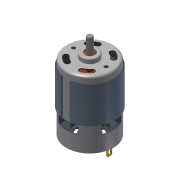
# Autodesk Inventor part: E Motor
Saved by Autodesk Inventor 2015 SP2 (Build 190223200, 223)
## iProperties
Created: 2015-09-01
Part Number: E Motor
Material: Iron, Cast
Document SubType Name: Modeling
Designer: Hassan
Density: 7.15 g/cm^3
Appearance: Iron Gray
Mass: 292.423 g
Surface Area: 270.91 cm^2
Volume: 40.8983 cm^3
Author: Hassan
Autodesk Inventor part; units mm, degrees
sketch "Sketch1" plane through (0, 0, 0) normal (0, 0, 1) x (1, 0, 0)
  circle A0 centre (0, 0) radius 21
  dimension "d3" = 42
  constraints: 1 centre point
  measures "d3" diameter of A0
extrude "Extrusion1" add sketch "Sketch1" along normal mid plane 59.5
sketch "Sketch2" plane through (0, 0, 29.75) normal (0, 0, 1) x (1, 0, 0)
  circle A0 centre (0, 0) radius 7.5
  dimension "d6" = 15
  constraints: 1 centre point, 1 coincident
  measures "d6" diameter of A0
extrude "Extrusion2" add sketch "Sketch2" along normal blind 4
sketch "Sketch3" plane through (0, 0, 33.75) normal (0, 0, 1) x (1, 0, 0)
  circle A0 centre (0, 0) radius 2.5
  dimension "d9" = 5
  constraints: 1 centre point, 1 coincident
  measures "d9" diameter of A0
extrude "Extrusion3" add sketch "Sketch3" along normal blind 13
sketch "Sketch4" plane through (0, 0, 29.75) normal (0, 0, 1) x (1, 0, 0)
  circle A0 centre (0, 0) radius 21 projected
  point P0 (-14.5, 0)
  point P1 (14.5, 0)
hole "Hole1" at (-14.5, 0, 29.75) at (14.5, 0, 29.75) direction (0, 0, -1) diameter 3.242 depth 3 thread size "M4x0.7" class "6H" standard "ANSI Metric M Profile"
fillet "Fillet1" radius 1 1 edges at (-2.5, 0, 46.75)
fillet "Fillet2" radius 1 1 edges at (-7.5, 0, 33.75)
fillet "Fillet3" radius 2 1 edges at (-21, 0, 29.75)
sketch "Sketch5" plane through (0, 0, -29.75) normal (0, 0, -1) x (-1, 0, 0)
  circle A0 centre (0, 0) radius 21 projected
  circle A1 centre (0, 0) radius 20.3
  circle A2 centre (0, 0) radius 14.5
  dimension "d25" = 29
  constraints: 2 centre point, 2 coincident
  measures "d25" diameter of A2
extrude "Extrusion4" cut sketch "Sketch5" against normal blind 1 contours A1
fillet "Fillet4" radius 1 1 edges at (14.5, 0, -29.75)
sketch "Sketch6" plane through (0, 0, -29.75) normal (0, 0, -1) x (-1, 0, 0)
  circle A0 centre (0, 0) radius 7.5
  dimension "d29" = 15
  constraints: 1 centre point, 1 coincident
  measures "d29" diameter of A0
extrude "Extrusion5" add sketch "Sketch6" along normal blind 4
sketch "Sketch7" plane through (0, 0, -33.75) normal (0, 0, -1) x (-1, 0, 0)
  circle A0 centre (0, 0) radius 5
  dimension "d32" = 10
  constraints: 1 centre point, 1 coincident
  measures "d32" diameter of A0
extrude "Extrusion6" add sketch "Sketch7" along normal blind 1
sketch "Sketch8" plane through (0, 0, -34.75) normal (0, 0, -1) x (-1, 0, 0)
  circle A0 centre (0, 0) radius 2.5
  dimension "d35" = 5
  constraints: 1 centre point, 1 coincident
  measures "d35" diameter of A0
extrude "Extrusion7" add sketch "Sketch8" along normal blind 1.8
fillet "Fillet5" radius 1 3 edges at (7.5, 0, -33.75) (5, 0, -34.75) (2.5, 0, -36.55)
sketch "Sketch9" plane through (0, 0, -28.75) normal (0, 0, -1) x (-1, 0, 0)
  circle A0 centre (0, 0) radius 20.3 projected
  line L0 (15.5, 0) -> (15.5, 4.54)
  line L1 (15.5, 4.54) -> (19.7858, 4.54)
  line L2 (15.5, 0) -> (15.5, -4.54)
  line L3 (15.5, -4.54) -> (19.7858, -4.54)
  arc A1 (19.7858, -4.54) -> (19.7858, 4.54) centre (0, 0) ccw
  constraints: 8 end point, 4 point on circle, 2 perpendicular, 1 centre point, 1 concentric, 1 vertical
extrude "Extrusion8" add sketch "Sketch9" along normal blind 1 contours A0 L3 L2 L0 L1 picked at (17.0236, 2.527)
sketch "Sketch10" plane through (0, 0, -29.75) normal (0, 0, -1) x (-1, 0, 0)
  line L0 (15.5, -4.54) -> (15.5, 4.54) projected
  line L1 (15.5, 0) -> (17.1, 0)
  line L2 (17.1, 0) -> (17.1, 2.35)
  line L3 (17.1, 2.35) -> (17.1, -2.35)
  line L4 (17.1, -2.35) -> (17.6, -2.35)
  line L5 (17.6, -2.35) -> (17.6, 2.35)
  line L6 (17.6, 2.35) -> (17.1, 2.35)
  point P0 (0, 0)
  dimension "d44" = 1.6
  dimension "d45" = 2.35
  dimension "d46" = 4.7
  dimension "d47" = 0.5
  constraints: 12 end point, 2 horizontal, 2 perpendicular, 1 midpoint, 1 point on line, 1 vertical
  measures "d44" distance of L1.start L1.end
  measures "d45" distance of L1.end L2.end
  measures "d46" distance of L2.end L3.end
  measures "d47" distance of L3.end L4.end
extrude "Extrusion9" add sketch "Sketch10" along normal blind 8.2
chamfer "Chamfer1" distance 1 angle 45 2 edges at (-17.35, -2.35, -37.95) (-17.35, 2.35, -37.95)
sketch "Sketch11" plane through (-17.6, -2.35, -29.75) normal (-1, 0, 0) x (0, 0, 1)
  line L0 (-5.8065, 2.35) -> (-4, 2.35) construction
  line L1 (-4, -4.15) -> (-4, 8.85) projected
  line L2 (-5.8065, 1.4883) -> (-4, 1.4883)
  line L3 (-4, 3.2117) -> (-5.8065, 3.2117)
  arc A0 (-5.8065, 3.2117) -> (-5.8065, 1.4883) centre (-5.8065, 2.35) ccw
  arc A1 (-4, 1.4883) -> (-4, 3.2117) centre (-4, 2.35) ccw
  line L4 (0, 4.7) -> (0, 3.7)
  line L5 (0, -5.15) -> (0, 9.85) projected
  line L6 (0, 3.7) -> (-1, 3.7)
  line L7 (-1, 3.7) -> (-1, 4.7)
  line L8 (0, 4.7) -> (-7.2, 4.7) projected
  line L9 (0, 0) -> (0, 1)
  line L10 (0, 1) -> (-1, 1)
  line L11 (-1, 1) -> (-1, 0)
  line L12 (0, 0) -> (-7.2, 0) projected
  point P0 (29.75, 2.35)
  point P1 (-4.9032, 2.35)
  dimension "d55" = 1
  dimension "d56" = 1
  dimension "d57" = 1
  dimension "d58" = 1
  constraints: 20 end point, 4 perpendicular, 4 point on circle, 4 point on line, 4 tangent, 2 centre point, 2 midpoint, 1 parallel
  measures "d55" distance of L4.start L4.end
  measures "d56" distance of L4.end L6.end
  measures "d57" distance of L9.start L9.end
  measures "d58" distance of L9.end L10.end
extrude "Extrusion10" cut sketch "Sketch11" against normal blind 0.5 contours L2 A0 L3 L1 | L1 A1 | L11 L10 L5 L12 | L8 L4 L6 L7
mirror "Mirror2" about plane through (0, 0, 0) normal (1, 0, 0) of "Extrusion10", "Chamfer1", "Extrusion9", "Extrusion8"
sketch "Sketch12" plane through (0, 0, 33.75) normal (0, 0, 1) x (1, 0, 0)
  circle A0 centre (0, 0) radius 2.5
  circle A1 centre (0, 0) radius 4.5
  dimension "d59" = 9
  constraints: 2 centre point, 2 coincident
  measures "d59" diameter of A1
extrude "Extrusion11" cut sketch "Sketch12" against normal blind 0.7
sketch "Sketch13" plane through (0, 0, -34.75) normal (0, 0, -1) x (-1, 0, 0)
  circle A0 centre (0, 0) radius 2.1875
  circle A1 centre (0, 0) radius 3.5
  dimension "d64" = 7
  constraints: 2 centre point, 2 coincident
  measures "d64" diameter of A1
extrude "Extrusion12" cut sketch "Sketch13" against normal blind 0.1
ref_plane "Work Plane1" through (0, 21, 0) normal (0, 1, 0) x (-1, 0, 0)
sketch "Sketch14" plane through (0, 21, 0) normal (0, 1, 0) x (-1, 0, 0)
  line L0 (-21, -29.75) -> (21, -29.75) projected
  line L1 (7.5, -8.75) -> (-7.5, -8.75)
  line L2 (-9, -10.25) -> (-9, -14.75)
  line L3 (-7.5, -16.25) -> (7.5, -16.25)
  line L4 (9, -14.75) -> (9, -10.25)
  line L5 (9, -8.75) -> (-9, -16.25) construction
  line L6 (-9, -8.75) -> (9, -16.25) construction
  arc A0 (7.5, -16.25) -> (9, -14.75) centre (7.5, -14.75) ccw
  arc A1 (9, -10.25) -> (7.5, -8.75) centre (7.5, -10.25) ccw
  arc A2 (-9, -14.75) -> (-7.5, -16.25) centre (-7.5, -14.75) ccw
  arc A3 (-7.5, -8.75) -> (-9, -10.25) centre (-7.5, -10.25) ccw
  point P0 (0, 0)
  point P1 (0, -12.5)
  constraints: 12 end point, 8 point on circle, 8 point on line, 8 tangent, 4 centre point, 3 equal radius, 2 midpoint, 2 parallel, 1 horizontal, 1 perpendicular
extrude "Extrusion13" cut sketch "Sketch14" against normal through all
pattern_circular "Circular Pattern1" count 2 over 90 about axis through (0, 0, -10) along (0, 0, 1) of "Extrusion13"
ref_plane "Work Plane2" through (0, 0, -28) normal (0, 0, 1) x (1, 0, 0)
sketch "Sketch15" plane through (0, 0, -28) normal (0, 0, 1) x (1, 0, 0)
  circle A0 centre (0, 0) radius 20.2
  dimension "d76" = 40.4
  constraints: 1 centre point, 1 coincident
  measures "d76" diameter of A0
extrude "Extrusion14" cut sketch "Sketch15" along normal blind 54.75
ref_plane "Work Plane3" through (0, 0, 26.75) normal (0, 0, 1) x (1, 0, 0)
sketch "Sketch16" plane through (0, 0, 26.75) normal (0, 0, 1) x (1, 0, 0)
  circle A0 centre (14.5, 0) radius 1.621 projected
  circle A1 centre (-14.5, 0) radius 1.621 projected
  circle A2 centre (0, 0) radius 19 projected
  circle A3 centre (14.5, 0) radius 2
  circle A4 centre (-14.5, 0) radius 2
  dimension "d80" = 4
  constraints: 2 centre point, 2 coincident
  measures "d80" diameter of A3
extrude "Extrusion15" cut sketch "Sketch16" along normal blind 2.2 contours A2
sketch "Sketch17" plane through (0, 0, 29.75) normal (0, 0, 1) x (1, 0, 0)
  arc A0 (13.5041, 11.1319) -> (7.3962, 15.8612) centre (0, 0) ccw
  arc A1 (9.8774, 8.1423) -> (5.4099, 11.6015) centre (0, 0) ccw
  arc A2 (9.8774, 8.1423) -> (13.5041, 11.1319) centre (11.6908, 9.6371) ccw
  arc A3 (7.3962, 15.8612) -> (5.4099, 11.6015) centre (6.403, 13.7313) ccw
  line L0 (0, 17.5008) -> (0, -16.5048)
  line L1 (17.6, 0) -> (-17.5008, 0)
  arc A4 (-7.3962, 15.8612) -> (-13.5041, 11.1319) centre (0, 0) ccw
  arc A5 (-5.4099, 11.6015) -> (-9.8774, 8.1423) centre (0, 0) ccw
  arc A6 (-13.5041, 11.1319) -> (-9.8774, 8.1423) centre (-11.6908, 9.6371) ccw
  arc A7 (-5.4099, 11.6015) -> (-7.3962, 15.8612) centre (-6.403, 13.7313) ccw
  arc A8 (7.3962, -15.8612) -> (13.5041, -11.1319) centre (0, 0) ccw
  arc A9 (5.4099, -11.6015) -> (9.8774, -8.1423) centre (0, 0) ccw
  arc A10 (13.5041, -11.1319) -> (9.8774, -8.1423) centre (11.6908, -9.6371) ccw
  arc A11 (5.4099, -11.6015) -> (7.3962, -15.8612) centre (6.403, -13.7313) ccw
  arc A12 (-13.5041, -11.1319) -> (-7.3962, -15.8612) centre (0, 0) ccw
  arc A13 (-9.8774, -8.1423) -> (-5.4099, -11.6015) centre (0, 0) ccw
  arc A14 (-9.8774, -8.1423) -> (-13.5041, -11.1319) centre (-11.6908, -9.6371) ccw
  arc A15 (-7.3962, -15.8612) -> (-5.4099, -11.6015) centre (-6.403, -13.7313) ccw
  constraints: 32 point on circle, 18 symmetric about line, 16 centre point, 4 end point, 4 tangent, 1 horizontal, 1 vertical, 12 other
extrude "Extrusion16" cut sketch "Sketch17" against normal blind 2.2
sketch "Sketch18" plane through (0, 0, -29.75) normal (0, 0, -1) x (-1, 0, 0)
  arc A0 (8.9348, 2.3941) -> (3.1637, 8.6922) centre (0, 0) ccw construction
  arc A1 (10.1422, 2.7176) -> (3.5912, 9.8668) centre (0, 0) ccw
  arc A2 (7.7274, 2.0706) -> (2.7362, 7.5175) centre (0, 0) ccw
  arc A3 (7.7274, 2.0706) -> (10.1422, 2.7176) centre (8.9348, 2.3941) ccw
  arc A4 (3.5912, 9.8668) -> (2.7362, 7.5175) centre (3.1637, 8.6922) ccw
  line L0 (0, 0) -> (8.9348, 2.3941) construction
  line L1 (0, 0) -> (9.25, 0) construction
  line L2 (0, 0) -> (3.1637, 8.6922) construction
  line L3 (0, 12.4664) -> (0, -11.4129)
  line L4 (11.5007, 0) -> (-11.1495, 0)
  arc A5 (-3.1637, 8.6922) -> (-8.9348, 2.3941) centre (0, 0) ccw construction
  arc A6 (-3.5912, 9.8668) -> (-10.1422, 2.7176) centre (0, 0) ccw
  arc A7 (-2.7362, 7.5175) -> (-7.7274, 2.0706) centre (0, 0) ccw
  arc A8 (-10.1422, 2.7176) -> (-7.7274, 2.0706) centre (-8.9348, 2.3941) ccw
  arc A9 (-2.7362, 7.5175) -> (-3.5912, 9.8668) centre (-3.1637, 8.6922) ccw
  arc A10 (3.1637, -8.6922) -> (8.9348, -2.3941) centre (0, 0) ccw construction
  arc A11 (3.5912, -9.8668) -> (10.1422, -2.7176) centre (0, 0) ccw
  arc A12 (2.7362, -7.5175) -> (7.7274, -2.0706) centre (0, 0) ccw
  arc A13 (10.1422, -2.7176) -> (7.7274, -2.0706) centre (8.9348, -2.3941) ccw
  arc A14 (2.7362, -7.5175) -> (3.5912, -9.8668) centre (3.1637, -8.6922) ccw
  arc A15 (-8.9348, -2.3941) -> (-3.1637, -8.6922) centre (0, 0) ccw construction
  arc A16 (-10.1422, -2.7176) -> (-3.5912, -9.8668) centre (0, 0) ccw
  arc A17 (-7.7274, -2.0706) -> (-2.7362, -7.5175) centre (0, 0) ccw
  arc A18 (-7.7274, -2.0706) -> (-10.1422, -2.7176) centre (-8.9348, -2.3941) ccw
  arc A19 (-3.5912, -9.8668) -> (-2.7362, -7.5175) centre (-3.1637, -8.6922) ccw
  dimension "d90" = 9.25
  dimension "d91" = 15
  dimension "d92" = 55
  dimension "d93" = 2.5
  constraints: 40 point on circle, 20 centre point, 18 symmetric about line, 10 end point, 4 tangent, 2 horizontal, 1 coincident, 1 equal length, 1 vertical, 15 other
  measures "d90" radius of A0
  measures "d91" angle of L1 L0
  measures "d92" angle of L0 L2
  measures "d93" diameter of A4
extrude "Extrusion17" cut sketch "Sketch18" against normal blind 2.2
sketch "Sketch19" plane through (0, 0, -28) normal (0, 0, 1) x (1, 0, 0)
  arc A0 (-3.5912, 9.8668) -> (-10.1422, 2.7176) centre (0, 0) ccw projected
  arc A1 (-2.7362, 7.5175) -> (-3.5912, 9.8668) centre (-3.1637, 8.6922) ccw projected
  arc A2 (-2.7362, 7.5175) -> (-7.7274, 2.0706) centre (0, 0) ccw projected
  arc A3 (-10.1422, 2.7176) -> (-7.7274, 2.0706) centre (-8.9348, 2.3941) ccw projected
  arc A4 (-7.7274, -2.0706) -> (-10.1422, -2.7176) centre (-8.9348, -2.3941) ccw projected
  arc A5 (-7.7274, -2.0706) -> (-2.7362, -7.5175) centre (0, 0) ccw projected
  arc A6 (-10.1422, -2.7176) -> (-3.5912, -9.8668) centre (0, 0) ccw projected
  arc A7 (-3.5912, -9.8668) -> (-2.7362, -7.5175) centre (-3.1637, -8.6922) ccw projected
  arc A8 (2.7362, -7.5175) -> (3.5912, -9.8668) centre (3.1637, -8.6922) ccw projected
  arc A9 (2.7362, -7.5175) -> (7.7274, -2.0706) centre (0, 0) ccw projected
  arc A10 (3.5912, -9.8668) -> (10.1422, -2.7176) centre (0, 0) ccw projected
  arc A11 (10.1422, -2.7176) -> (7.7274, -2.0706) centre (8.9348, -2.3941) ccw projected
  arc A12 (7.7274, 2.0706) -> (10.1422, 2.7176) centre (8.9348, 2.3941) ccw projected
  arc A13 (7.7274, 2.0706) -> (2.7362, 7.5175) centre (0, 0) ccw projected
  arc A14 (10.1422, 2.7176) -> (3.5912, 9.8668) centre (0, 0) ccw projected
  arc A15 (3.5912, 9.8668) -> (2.7362, 7.5175) centre (3.1637, 8.6922) ccw projected
  circle A16 centre (0, 0) radius 12.663
  constraints: 1 centre point
extrude "Extrusion18" cut sketch "Sketch19" against normal blind 0.6
sketch "Sketch20" plane through (0, 0, 0) normal (0, 0, 1) x (1, 0, 0)
  circle A0 centre (0, 0) radius 14.5
  circle A1 centre (0, 0) radius 20.2 projected
  arc A2 (-13.5041, -11.1319) -> (13.5041, -11.1319) centre (0, 0) ccw construction
  arc A3 (-15.5868, -12.8488) -> (15.5868, -12.8488) centre (0, 0) ccw
  arc A4 (-11.4214, -9.415) -> (11.4214, -9.415) centre (0, 0) ccw
  arc A5 (-11.4214, -9.415) -> (-15.5868, -12.8488) centre (-13.5041, -11.1319) ccw
  arc A6 (15.5868, -12.8488) -> (11.4214, -9.415) centre (13.5041, -11.1319) ccw
  line L0 (3.7214, 0) -> (-6.1083, 0)
  arc A7 (15.5868, 12.8488) -> (-15.5868, 12.8488) centre (0, 0) ccw
  arc A8 (11.4214, 9.415) -> (-11.4214, 9.415) centre (0, 0) ccw
  arc A9 (-15.5868, 12.8488) -> (-11.4214, 9.415) centre (-13.5041, 11.1319) ccw
  arc A10 (11.4214, 9.415) -> (15.5868, 12.8488) centre (13.5041, 11.1319) ccw
  dimension "d98" = 29
  constraints: 18 point on circle, 10 centre point, 6 symmetric about line, 4 tangent, 2 end point, 1 coincident, 1 concentric, 1 horizontal, 4 other
  measures "d98" diameter of A0
extrude "Extrusion19" add sketch "Sketch20" along normal blind 20 contours A0 | A10 A8 A9 A1 | A1 A5 A4 A6
sketch "Sketch21" plane through (0, 0, 0) normal (0, 0, -1) x (-1, 0, 0)
  circle A0 centre (0, 0) radius 2.5
  constraints: 1 centre point, 1 coincident
extrude "Extrusion20" add sketch "Sketch21" along normal mid plane 66
sketch "Sketch22" plane through (0, 0, 0) normal (0, 0, -1) x (-1, 0, 0)
  circle A0 centre (0, 0) radius 11.6
  dimension "d103" = 23.2
  constraints: 1 centre point, 1 coincident
  measures "d103" diameter of A0
extrude "Extrusion21" add sketch "Sketch22" along normal blind 8.75
sketch "Sketch23" plane through (0, 0, -28.6) normal (0, 0, 1) x (1, 0, 0)
  circle A0 centre (0, 0) radius 21
  line L0 (1.5, 3.848) -> (1.5, 6.3246)
  line L1 (-1.5, 6.3246) -> (-1.5, 3.848)
  line L2 (-0.7498, 6.3246) -> (-0.7498, 13.4792)
  arc A1 (14.0458, 2.4156) -> (-0.0019, 14.229) centre (0.0369, 0.0161) ccw
  arc A2 (12.7502, 0.0009) -> (0.7502, 12.7093) centre (0.0369, 0.0161) ccw
  arc A3 (-0.0019, 14.229) -> (-0.7497, 13.4792) centre (0.0002, 13.4792) ccw
  arc A4 (0.0737, 13.4792) -> (0.0002, 13.4792) centre (0.0369, 0.0161) ccw construction
  line L3 (-0.7498, 13.4792) -> (-0.7497, 13.4792)
  line L4 (0.7502, 13.4792) -> (0.7502, 13.4603)
  line L5 (0.7502, 12.7093) -> (0.7502, 6.3246)
  line L6 (0.0002, 13.4792) -> (0.0737, 13.4792)
  line L7 (0.7498, 13.4792) -> (0.7502, 13.4792)
  line L8 (1.5, 6.3246) -> (0.7502, 6.3246)
  line L9 (-0.7498, 6.3246) -> (-1.5, 6.3246)
  arc A5 (1.5, 3.848) -> (-1.5, 3.848) centre (0, 0) ccw
  line L10 (14.0458, 2.4156) -> (19.5458, 2.4156)
  line L11 (19.5458, 2.4156) -> (19.5458, -2.5844)
  line L12 (19.5458, -2.5844) -> (12.7502, -2.5844)
  line L13 (12.7502, -2.5844) -> (12.7502, 0.0009)
  line L14 (-1.5, -3.848) -> (-1.5, -6.3246)
  line L15 (1.5, -6.3246) -> (1.5, -3.848)
  line L16 (0.7498, -6.3246) -> (0.7498, -13.4792)
  arc A6 (-14.0458, -2.4156) -> (0.0019, -14.229) centre (-0.0369, -0.0161) ccw
  arc A7 (-12.7502, -0.0009) -> (-0.7502, -12.7093) centre (-0.0369, -0.0161) ccw
  arc A8 (0.0019, -14.229) -> (0.7497, -13.4792) centre (-0.0002, -13.4792) ccw
  arc A9 (-0.0737, -13.4792) -> (-0.0002, -13.4792) centre (-0.0369, -0.0161) ccw construction
  line L17 (0.7498, -13.4792) -> (0.7497, -13.4792)
  line L18 (-0.7502, -13.4792) -> (-0.7502, -13.4603)
  line L19 (-0.7502, -12.7093) -> (-0.7502, -6.3246)
  line L20 (-0.0002, -13.4792) -> (-0.0737, -13.4792)
  line L21 (-0.7498, -13.4792) -> (-0.7502, -13.4792)
  line L22 (-1.5, -6.3246) -> (-0.7502, -6.3246)
  line L23 (0.7498, -6.3246) -> (1.5, -6.3246)
  arc A10 (-1.5, -3.848) -> (1.5, -3.848) centre (0, 0) ccw
  line L24 (-14.0458, -2.4156) -> (-19.5458, -2.4156)
  line L25 (-19.5458, -2.4156) -> (-19.5458, 2.5844)
  line L26 (-19.5458, 2.5844) -> (-12.7502, 2.5844)
  line L27 (-12.7502, 2.5844) -> (-12.7502, -0.0009)
  constraints: 56 end point, 20 point on circle, 12 centre point, 6 parallel, 6 perpendicular, 4 tangent, 1 horizontal
sketch "Sketch24" plane through (0, 0, 0) normal (1, 0, 0) x (0, 1, 0)
  line L0 (0, 0) -> (0, -28)
  line L1 (-8.795, -12.4742) -> (-8.795, -12.0628)
  line L2 (8.795, -11.5198) -> (8.795, -12.9742)
  arc A0 (-8.2538, -11.5645) -> (-8.795, -12.0628) centre (-8.295, -12.0628) ccw
  arc A1 (-8.795, -12.4742) -> (-8.295, -12.9742) centre (-8.295, -12.4742) ccw
  line L3 (-7.8889, -12.9742) -> (-8.295, -12.9742)
  line L4 (-8.2538, -11.5645) -> (-2.5, -11.5645)
  line L5 (-2.5, -12.9742) -> (-2.5, -11.5645)
  line L6 (-2.5, -12.9742) -> (-2.5, -15.6196)
  arc A2 (-7.8889, -12.9742) -> (-2.5, -15.6196) centre (-2.2288, -8.2555) ccw
  arc A3 (-7.8889, -8.75) -> (-2.5, -11.2897) centre (-0.1389, 0.7073) ccw
  line L7 (-7.8889, -8.75) -> (-2.5, -8.75)
  line L8 (-2.5, -8.75) -> (-2.5, -11.2897)
  point P0 (0, -12.247)
  constraints: 18 end point, 8 point on circle, 4 centre point, 3 tangent, 2 horizontal, 2 perpendicular, 2 vertical, 1 equal radius, 1 parallel, 1 point on line
revolve "Revolution1" add sketch "Sketch24" angle 360 about axis through (0, 0, 0) along (0, 0, -1)
extrude "Extrusion22" add sketch "Sketch23" along normal blind 5 contours A5 L1 L9 L2 A3 A1 L10 L11 L12 L13 A2 L5 L8 L0 | A10 L15 L23 L16 A8 A6 L24 L25 L26 L27 A7 L19 L22 L14
sketch "Sketch25" plane through (0, 0, -28.6) normal (0, 0, 1) x (1, 0, 0)
  circle A0 centre (0, 0) radius 4.1
  dimension "d119" = 8.2
  constraints: 1 centre point, 1 coincident
  measures "d119" diameter of A0
extrude "Extrusion23" add sketch "Sketch25" along normal blind 12.25
ref_plane "Work Plane4" through (0, 0, -8) normal (0, 0, 1) x (1, 0, 0)
sketch "Sketch27" plane through (0, 0, -8) normal (0, 0, 1) x (1, 0, 0)
  arc A0 (3.484, -20.709) -> (-3.484, -20.709) centre (0, 0) ccw
  arc A1 (3.6499, -21.6951) -> (-3.6499, -21.6951) centre (0, 0) ccw
  line L0 (3.484, -20.709) -> (3.6499, -21.6951)
  line L1 (-3.484, -20.709) -> (-3.6499, -21.6951)
  constraints: 4 end point, 4 point on circle, 2 centre point, 1 coincident
extrude "Extrusion25" add sketch "Sketch27" along normal blind 32
body "Solid1"
